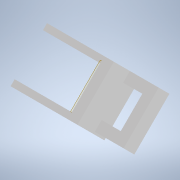
# Autodesk Inventor part: StrapHolder
Saved by Autodesk Inventor 2022 (Build 260153000, 153)
## iProperties
Created: 2022-02-23
Part Number: StrapHolder
Material: Generic
Document SubType Name: Modeling
Designer: siwat
Density: 1 g/cm^3
Appearance: Default
Author: siwat
Autodesk Inventor part; units mm, degrees
ref_plane "YZ Plane" through (0, 0, 0) normal (1, 0, 0) x (0, 1, 0)
ref_plane "XZ Plane" through (0, 0, 0) normal (0, 1, 0) x (-1, 0, 0)
ref_plane "XY Plane" through (0, 0, 0) normal (0, 0, 1) x (1, 0, 0)
ref_plane "Work Plane1" through (400, -8.5282, -0.75) normal (1, 0, 0) x (0, 0.7071068, -0.7071068)
sketch "Sketch1" plane through (400, -8.5282, -0.75) normal (1, 0, 0) x (0, 0.7071068, -0.7071068)
  line L0 (-10.9826, 10.0209) -> (10.0174, 10.0209)
  line L1 (10.0174, 10.0209) -> (10.0174, -9.9791)
  line L2 (10.0174, -9.9791) -> (-10.9826, -9.9791)
  line L3 (-10.9826, -9.9791) -> (-10.9826, 10.0209)
  line L4 (10.0174, 10.0209) -> (13.0174, 10.0209)
  line L5 (13.0174, 10.0209) -> (13.0174, -9.9791)
  line L6 (13.0174, -9.9791) -> (10.0174, -9.9791)
  line L7 (10.0174, -9.9791) -> (10.0174, 10.0209)
  line L8 (-10.9826, 10.0209) -> (-13.9826, 10.0209)
  line L9 (-13.9826, 10.0209) -> (-13.9826, -9.9791)
  line L10 (-13.9826, -9.9791) -> (-10.9826, -9.9791)
  line L11 (-10.9826, -9.9791) -> (-10.9826, 10.0209)
  point P0 (5.5, 6.5607)
  point P1 (10.0174, -9.9791)
  point P2 (-10.9826, -9.9791)
  dimension "d0" = 21
  dimension "d1" = 20
  dimension "d2" = 3
  dimension "d3" = 20
  dimension "d4" = 3
  dimension "d5" = 20
  constraints: 24 end point, 6 parallel, 3 horizontal, 3 perpendicular
  measures "d0" distance of L1.end L2.end
  measures "d1" distance of L0.end L1.end
  measures "d2" distance of L5.end L6.end
  measures "d3" distance of L4.end L5.end
  measures "d4" distance of L10.end L9.end
  measures "d5" distance of L9.end L8.end
extrude "Extrusion1" add sketch "Sketch1" against normal blind 30 contours L3 L10 L9 L8 | L4 L5 L6 L1
sketch "Sketch2" plane through (400, -8.5282, -0.75) normal (1, 0, 0) x (0, -0.7071068, -0.7071068)
  line L0 (-10.0209, -13.9826) -> (-10.0209, -10.9826) projected
  line L1 (9.9791, 13.0174) -> (9.9791, 10.0174) projected
  line L2 (-10.0209, -13.9826) -> (9.9791, -13.9826)
  line L3 (9.9791, -13.9826) -> (9.9791, 13.0174)
  line L4 (9.9791, 13.0174) -> (-10.0209, 13.0174)
  line L5 (-10.0209, 13.0174) -> (-10.0209, -13.9826)
  point P0 (-6.5607, 5.5)
  constraints: 8 end point, 2 parallel, 1 horizontal, 1 perpendicular
extrude "Extrusion2" add sketch "Sketch2" along normal blind 5
sketch "Sketch3" plane through (405, -6.3798, -17.011) normal (0, -0.7071068, -0.7071068) x (-1, 0, 0)
  line L0 (35, 0) -> (0, 0) projected
  line L1 (0, 0) -> (-15, 0)
  line L2 (-15, 0) -> (-15, -26)
  line L3 (-15, -26) -> (0, -26)
  line L4 (0, -26) -> (0, 0)
  line L5 (-10.0102, -5) -> (0, -5)
  line L6 (0, -5) -> (0, -21)
  line L7 (0, -21) -> (-10.0102, -21)
  line L8 (-10.0102, -21) -> (-10.0102, -5)
  point P0 (405, -7.5174)
  point P1 (0, -21)
  point P2 (0, -5)
  dimension "d10" = 15
  dimension "d11" = 26
  dimension "d12" = 0
  dimension "d13" = 5
  dimension "d14" = 16
  constraints: 16 end point, 4 parallel, 2 horizontal, 2 perpendicular
  measures "d10" distance of L3.end L2.end
  measures "d11" distance of L2.end L1.end
  measures "d12" distance between parallel lines of L4 L6
  measures "d13" distance between parallel lines of L3 L7
  measures "d14" distance of L7.end L5.start
extrude "Extrusion3" add sketch "Sketch3" against normal blind 8 contours L4 L5 L8 L7 L3 L2 L1
sketch "Sketch4" plane through (370, -11.3295, 16.223) normal (0, -0.7071068, 0.7071068) x (1, 0, 0)
  circle A0 centre (15, -10) radius 2.75
  line L0 (0, -20) -> (50, -20) projected
  line L1 (0, -20) -> (0, 0) projected
  point P0 (-370, -3.4602)
  dimension "d17" = 5.5
  dimension "d18" = 10
  dimension "d19" = 15
  constraints: 1 centre point
  measures "d17" diameter of A0
  measures "d18" distance from line of L0 A0.centre
  measures "d19" distance from line of A0.centre L1
extrude "Extrusion4" cut sketch "Sketch4" against normal through all
sketch "Sketch5" plane through (370, -11.3295, 16.223) normal (0, -0.7071068, 0.7071068) x (1, 0, 0)
  circle A0 centre (15, -10) radius 2.75 projected
  circle A1 centre (15, -10) radius 5.75
  point P0 (-370, -3.4602)
  dimension "d22" = 11.5
  constraints: 1 centre point, 1 coincident
  measures "d22" diameter of A1
extrude "Extrusion5" cut sketch "Sketch5" against normal blind 1 contours A0 | A1
sketch "Sketch6" plane through (405, 7.7624, -2.8688) normal (0, 0.7071068, -0.7071068) x (-1, 0, 0)
  circle A0 centre (20, -10) radius 2.75 projected
  circle A1 centre (20, -10) radius 5.75
  point P0 (405, -3.4602)
  dimension "d25" = 11.5
  constraints: 1 centre point, 1 coincident
  measures "d25" diameter of A1
extrude "Extrusion6" cut sketch "Sketch6" against normal blind 1
equation "\"d14\" = d11 - 2 * d13"
body "Solid1"
